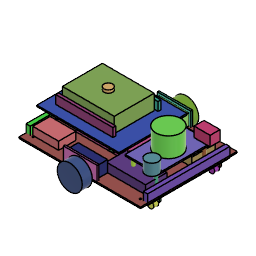
Vibration_Aware_AMR_Concept_v02 (Autodesk Fusion 360 design; units mm, degrees)
part number: 2026-07-23-00-14-06-650
part number: 2026-07-23-00-14-06-952
part number: 2026-07-23-00-14-07-093
part number: 2026-07-23-00-14-07-134
part number: 2026-07-23-00-14-07-172
part number: 2026-07-23-00-14-07-216
part number: 2026-07-23-00-14-07-265
part number: 2026-07-23-00-14-07-312
part number: 2026-07-23-00-14-07-363
part number: 2026-07-23-00-14-07-419
part number: 2026-07-23-00-14-07-476
part number: 2026-07-23-00-14-07-530
part number: 2026-07-23-00-14-07-582
part number: 2026-07-23-00-14-07-638
part number: 2026-07-23-00-14-07-701
part number: 2026-07-23-00-14-07-770
part number: 2026-07-23-00-14-07-834
part number: 2026-07-23-00-14-07-909
part number: 2026-07-23-00-14-07-976
part number: 2026-07-23-00-14-08-046
part number: 2026-07-23-00-14-08-123
part number: 2026-07-23-00-14-08-206
part number: 2026-07-23-00-14-08-287
part number: 2026-07-23-00-14-08-375
part number: 2026-07-23-00-14-08-464
part number: 2026-07-23-00-14-08-554
part number: 2026-07-23-00-14-08-651
part number: 2026-07-23-00-14-08-745
part number: 2026-07-23-00-14-08-842
part number: 2026-07-23-00-14-08-938
part number: 2026-07-23-00-14-09-021
part number: 2026-07-23-00-14-09-105
part number: 2026-07-23-00-14-09-197
part number: 2026-07-23-00-14-09-296
part number: 2026-07-23-00-14-09-389
part number: 2026-07-23-00-14-09-480
part number: 2026-07-23-00-14-09-570
part number: 2026-07-23-00-14-09-668
part number: 2026-07-23-00-14-09-762
part number: 2026-07-23-00-14-09-860
part number: 2026-07-23-00-14-09-959
part number: 2026-07-23-00-14-10-055
part number: 2026-07-23-00-14-10-157
Autodesk Fusion 360 part; units mm, degrees
sketch "00_Chassis_Base_Plate_Footprint" plane through (0, 0, 0) normal (0, 0, 1) x (1, 0, 0) in component "00_Chassis_Base_Plate"
  line L0 (-170, -135) -> (170, -135)
  line L1 (170, -135) -> (170, 135)
  line L2 (170, 135) -> (-170, 135)
  line L3 (-170, 135) -> (-170, -135)
extrude "00_Chassis_Base_Plate_Extrude" add sketch "00_Chassis_Base_Plate_Footprint" along normal blind 4 makes body 1 in component "00_Chassis_Base_Plate"
sketch "Mounting_Hole_Grid" plane through (0, 0, 0) normal (0, 0, 1) x (1, 0, 0) in component "00_Chassis_Base_Plate"
  circle A0 centre (-150, -115) radius 2.5
  circle A1 centre (-150, 115) radius 2.5
  circle A2 centre (150, -115) radius 2.5
  circle A3 centre (150, 115) radius 2.5
  circle A4 centre (-100, -85) radius 2.5
  circle A5 centre (-100, 85) radius 2.5
  circle A6 centre (0, -85) radius 2.5
  circle A7 centre (0, 85) radius 2.5
  circle A8 centre (100, -85) radius 2.5
  circle A9 centre (100, 85) radius 2.5
extrude "Mounting_Holes_Cut" cut sketch "Mounting_Hole_Grid" along normal blind 4 bodies 1 in component "00_Chassis_Base_Plate"
sketch "01_Left_Drive_Wheel_Profile" plane through (0, 0, 0) normal (0, 1, 0) x (1, 0, 0) in component "01_Left_Drive_Wheel"
  circle A0 centre (0, 0) radius 35
extrude "01_Left_Drive_Wheel_Extrude" add sketch "01_Left_Drive_Wheel_Profile" along normal blind 28 separate body makes body 2 in component "01_Left_Drive_Wheel"
sketch "02_Right_Drive_Wheel_Profile" plane through (0, 0, 0) normal (0, 1, 0) x (1, 0, 0) in component "02_Right_Drive_Wheel"
  circle A0 centre (0, 0) radius 35
extrude "02_Right_Drive_Wheel_Extrude" add sketch "02_Right_Drive_Wheel_Profile" along normal blind 28 separate body makes body 3 in component "02_Right_Drive_Wheel"
sketch "03_Left_Wheel_Guard_Footprint" plane through (0, 0, 0) normal (0, 0, 1) x (1, 0, 0) in component "03_Left_Wheel_Guard"
  line L0 (-47, -2.5) -> (47, -2.5)
  line L1 (47, -2.5) -> (47, 2.5)
  line L2 (47, 2.5) -> (-47, 2.5)
  line L3 (-47, 2.5) -> (-47, -2.5)
extrude "03_Left_Wheel_Guard_Extrude" add sketch "03_Left_Wheel_Guard_Footprint" along normal blind 42 separate body makes body 4 in component "03_Left_Wheel_Guard"
sketch "04_Right_Wheel_Guard_Footprint" plane through (0, 0, 0) normal (0, 0, 1) x (1, 0, 0) in component "04_Right_Wheel_Guard"
  line L0 (-47, -2.5) -> (47, -2.5)
  line L1 (47, -2.5) -> (47, 2.5)
  line L2 (47, 2.5) -> (-47, 2.5)
  line L3 (-47, 2.5) -> (-47, -2.5)
extrude "04_Right_Wheel_Guard_Extrude" add sketch "04_Right_Wheel_Guard_Footprint" along normal blind 42 separate body makes body 5 in component "04_Right_Wheel_Guard"
sketch "05_Rear_Caster_Soft_Tread_Profile" plane through (0, 0, 0) normal (0, 1, 0) x (1, 0, 0) in component "05_Rear_Caster_Soft_Tread"
  circle A0 centre (0, 0) radius 20
extrude "05_Rear_Caster_Soft_Tread_Extrude" add sketch "05_Rear_Caster_Soft_Tread_Profile" along normal blind 24 separate body makes body 6 in component "05_Rear_Caster_Soft_Tread"
sketch "06_Rear_Caster_Fork_Left_Footprint" plane through (0, 0, 0) normal (0, 0, 1) x (1, 0, 0) in component "06_Rear_Caster_Fork_Left"
  line L0 (-21, -2) -> (21, -2)
  line L1 (21, -2) -> (21, 2)
  line L2 (21, 2) -> (-21, 2)
  line L3 (-21, 2) -> (-21, -2)
extrude "06_Rear_Caster_Fork_Left_Extrude" add sketch "06_Rear_Caster_Fork_Left_Footprint" along normal blind 26 separate body makes body 7 in component "06_Rear_Caster_Fork_Left"
sketch "07_Rear_Caster_Fork_Right_Footprint" plane through (0, 0, 0) normal (0, 0, 1) x (1, 0, 0) in component "07_Rear_Caster_Fork_Right"
  line L0 (-21, -2) -> (21, -2)
  line L1 (21, -2) -> (21, 2)
  line L2 (21, 2) -> (-21, 2)
  line L3 (-21, 2) -> (-21, -2)
extrude "07_Rear_Caster_Fork_Right_Extrude" add sketch "07_Rear_Caster_Fork_Right_Footprint" along normal blind 26 separate body makes body 8 in component "07_Rear_Caster_Fork_Right"
sketch "08_Rear_Caster_Fork_Bridge_Footprint" plane through (0, 0, 0) normal (0, 0, 1) x (1, 0, 0) in component "08_Rear_Caster_Fork_Bridge"
  line L0 (-14, -19) -> (14, -19)
  line L1 (14, -19) -> (14, 19)
  line L2 (14, 19) -> (-14, 19)
  line L3 (-14, 19) -> (-14, -19)
extrude "08_Rear_Caster_Fork_Bridge_Extrude" add sketch "08_Rear_Caster_Fork_Bridge_Footprint" along normal blind 5 separate body makes body 9 in component "08_Rear_Caster_Fork_Bridge"
sketch "09_Rear_Caster_Swivel_Stem_Profile" plane through (0, 0, 0) normal (0, 0, 1) x (1, 0, 0) in component "09_Rear_Caster_Swivel_Stem"
  circle A0 centre (0, 0) radius 8
extrude "09_Rear_Caster_Swivel_Stem_Extrude" add sketch "09_Rear_Caster_Swivel_Stem_Profile" along normal blind 10 separate body makes body 10 in component "09_Rear_Caster_Swivel_Stem"
sketch "10_Front_AntiTip_Roller_Left_Profile" plane through (0, 0, 0) normal (0, 1, 0) x (1, 0, 0) in component "10_Front_AntiTip_Roller_Left"
  circle A0 centre (0, 0) radius 10
extrude "10_Front_AntiTip_Roller_Left_Extrude" add sketch "10_Front_AntiTip_Roller_Left_Profile" along normal blind 14 separate body makes body 11 in component "10_Front_AntiTip_Roller_Left"
sketch "11_Front_AntiTip_Roller_Right_Profile" plane through (0, 0, 0) normal (0, 1, 0) x (1, 0, 0) in component "11_Front_AntiTip_Roller_Right"
  circle A0 centre (0, 0) radius 10
extrude "11_Front_AntiTip_Roller_Right_Extrude" add sketch "11_Front_AntiTip_Roller_Right_Profile" along normal blind 14 separate body makes body 12 in component "11_Front_AntiTip_Roller_Right"
sketch "12_Front_AntiTip_Bracket_Left_Footprint" plane through (0, 0, 0) normal (0, 0, 1) x (1, 0, 0) in component "12_Front_AntiTip_Bracket_Left"
  line L0 (-17, -2.5) -> (17, -2.5)
  line L1 (17, -2.5) -> (17, 2.5)
  line L2 (17, 2.5) -> (-17, 2.5)
  line L3 (-17, 2.5) -> (-17, -2.5)
extrude "12_Front_AntiTip_Bracket_Left_Extrude" add sketch "12_Front_AntiTip_Bracket_Left_Footprint" along normal blind 18 separate body makes body 13 in component "12_Front_AntiTip_Bracket_Left"
sketch "13_Front_AntiTip_Bracket_Right_Footprint" plane through (0, 0, 0) normal (0, 0, 1) x (1, 0, 0) in component "13_Front_AntiTip_Bracket_Right"
  line L0 (-17, -2.5) -> (17, -2.5)
  line L1 (17, -2.5) -> (17, 2.5)
  line L2 (17, 2.5) -> (-17, 2.5)
  line L3 (-17, 2.5) -> (-17, -2.5)
extrude "13_Front_AntiTip_Bracket_Right_Extrude" add sketch "13_Front_AntiTip_Bracket_Right_Footprint" along normal blind 18 separate body makes body 14 in component "13_Front_AntiTip_Bracket_Right"
sketch "20_Left_Gearmotor_Envelope_Footprint" plane through (0, 0, 0) normal (0, 0, 1) x (1, 0, 0) in component "20_Left_Gearmotor_Envelope"
  line L0 (-41, -16) -> (41, -16)
  line L1 (41, -16) -> (41, 16)
  line L2 (41, 16) -> (-41, 16)
  line L3 (-41, 16) -> (-41, -16)
extrude "20_Left_Gearmotor_Envelope_Extrude" add sketch "20_Left_Gearmotor_Envelope_Footprint" along normal blind 32 separate body makes body 15 in component "20_Left_Gearmotor_Envelope"
sketch "21_Right_Gearmotor_Envelope_Footprint" plane through (0, 0, 0) normal (0, 0, 1) x (1, 0, 0) in component "21_Right_Gearmotor_Envelope"
  line L0 (-41, -16) -> (41, -16)
  line L1 (41, -16) -> (41, 16)
  line L2 (41, 16) -> (-41, 16)
  line L3 (-41, 16) -> (-41, -16)
extrude "21_Right_Gearmotor_Envelope_Extrude" add sketch "21_Right_Gearmotor_Envelope_Footprint" along normal blind 32 separate body makes body 16 in component "21_Right_Gearmotor_Envelope"
sketch "22_Low_Central_Battery_12V_Envelope_Footprint" plane through (0, 0, 0) normal (0, 0, 1) x (1, 0, 0) in component "22_Low_Central_Battery_12V_Envelope"
  line L0 (-72.5, -43) -> (72.5, -43)
  line L1 (72.5, -43) -> (72.5, 43)
  line L2 (72.5, 43) -> (-72.5, 43)
  line L3 (-72.5, 43) -> (-72.5, -43)
extrude "22_Low_Central_Battery_12V_Envelope_Extrude" add sketch "22_Low_Central_Battery_12V_Envelope_Footprint" along normal blind 42 separate body makes body 17 in component "22_Low_Central_Battery_12V_Envelope"
sketch "23_Battery_Retention_Crossbar_Footprint" plane through (0, 0, 0) normal (0, 0, 1) x (1, 0, 0) in component "23_Battery_Retention_Crossbar"
  line L0 (-6, -50) -> (6, -50)
  line L1 (6, -50) -> (6, 50)
  line L2 (6, 50) -> (-6, 50)
  line L3 (-6, 50) -> (-6, -50)
extrude "23_Battery_Retention_Crossbar_Extrude" add sketch "23_Battery_Retention_Crossbar_Footprint" along normal blind 12 separate body makes body 18 in component "23_Battery_Retention_Crossbar"
sketch "24_Raspberry_Pi_4_Envelope_Footprint" plane through (0, 0, 0) normal (0, 0, 1) x (1, 0, 0) in component "24_Raspberry_Pi_4_Envelope"
  line L0 (-45, -32.5) -> (45, -32.5)
  line L1 (45, -32.5) -> (45, 32.5)
  line L2 (45, 32.5) -> (-45, 32.5)
  line L3 (-45, 32.5) -> (-45, -32.5)
extrude "24_Raspberry_Pi_4_Envelope_Extrude" add sketch "24_Raspberry_Pi_4_Envelope_Footprint" along normal blind 24 separate body makes body 19 in component "24_Raspberry_Pi_4_Envelope"
sketch "25_Arduino_Mega_Envelope_Footprint" plane through (0, 0, 0) normal (0, 0, 1) x (1, 0, 0) in component "25_Arduino_Mega_Envelope"
  line L0 (-55, -30) -> (55, -30)
  line L1 (55, -30) -> (55, 30)
  line L2 (55, 30) -> (-55, 30)
  line L3 (-55, 30) -> (-55, -30)
extrude "25_Arduino_Mega_Envelope_Extrude" add sketch "25_Arduino_Mega_Envelope_Footprint" along normal blind 24 separate body makes body 20 in component "25_Arduino_Mega_Envelope"
sketch "26_Motor_Driver_Envelope_Footprint" plane through (0, 0, 0) normal (0, 0, 1) x (1, 0, 0) in component "26_Motor_Driver_Envelope"
  line L0 (-36, -26) -> (36, -26)
  line L1 (36, -26) -> (36, 26)
  line L2 (36, 26) -> (-36, 26)
  line L3 (-36, 26) -> (-36, -26)
extrude "26_Motor_Driver_Envelope_Extrude" add sketch "26_Motor_Driver_Envelope_Footprint" along normal blind 22 separate body makes body 21 in component "26_Motor_Driver_Envelope"
sketch "27_Power_Distribution_Envelope_Footprint" plane through (0, 0, 0) normal (0, 0, 1) x (1, 0, 0) in component "27_Power_Distribution_Envelope"
  line L0 (-36, -24) -> (36, -24)
  line L1 (36, -24) -> (36, 24)
  line L2 (36, 24) -> (-36, 24)
  line L3 (-36, 24) -> (-36, -24)
extrude "27_Power_Distribution_Envelope_Extrude" add sketch "27_Power_Distribution_Envelope_Footprint" along normal blind 22 separate body makes body 22 in component "27_Power_Distribution_Envelope"
sketch "28_Chassis_IMU_Envelope_Profile" plane through (0, 0, 0) normal (0, 0, 1) x (1, 0, 0) in component "28_Chassis_IMU_Envelope"
  circle A0 centre (0, 0) radius 12
extrude "28_Chassis_IMU_Envelope_Extrude" add sketch "28_Chassis_IMU_Envelope_Profile" along normal blind 8 separate body makes body 23 in component "28_Chassis_IMU_Envelope"
sketch "30_Sensor_Bridge_Standoff_1_Profile" plane through (0, 0, 0) normal (0, 0, 1) x (1, 0, 0) in component "30_Sensor_Bridge_Standoff_1"
  circle A0 centre (0, 0) radius 5
extrude "30_Sensor_Bridge_Standoff_1_Extrude" add sketch "30_Sensor_Bridge_Standoff_1_Profile" along normal blind 42 separate body makes body 24 in component "30_Sensor_Bridge_Standoff_1"
sketch "30_Sensor_Bridge_Standoff_2_Profile" plane through (0, 0, 0) normal (0, 0, 1) x (1, 0, 0) in component "30_Sensor_Bridge_Standoff_2"
  circle A0 centre (0, 0) radius 5
extrude "30_Sensor_Bridge_Standoff_2_Extrude" add sketch "30_Sensor_Bridge_Standoff_2_Profile" along normal blind 42 separate body makes body 25 in component "30_Sensor_Bridge_Standoff_2"
sketch "30_Sensor_Bridge_Standoff_3_Profile" plane through (0, 0, 0) normal (0, 0, 1) x (1, 0, 0) in component "30_Sensor_Bridge_Standoff_3"
  circle A0 centre (0, 0) radius 5
extrude "30_Sensor_Bridge_Standoff_3_Extrude" add sketch "30_Sensor_Bridge_Standoff_3_Profile" along normal blind 42 separate body makes body 26 in component "30_Sensor_Bridge_Standoff_3"
sketch "30_Sensor_Bridge_Standoff_4_Profile" plane through (0, 0, 0) normal (0, 0, 1) x (1, 0, 0) in component "30_Sensor_Bridge_Standoff_4"
  circle A0 centre (0, 0) radius 5
extrude "30_Sensor_Bridge_Standoff_4_Extrude" add sketch "30_Sensor_Bridge_Standoff_4_Profile" along normal blind 42 separate body makes body 27 in component "30_Sensor_Bridge_Standoff_4"
sketch "34_Rigid_Sensor_Bridge_Footprint" plane through (0, 0, 0) normal (0, 0, 1) x (1, 0, 0) in component "34_Rigid_Sensor_Bridge"
  line L0 (-46, -75) -> (46, -75)
  line L1 (46, -75) -> (46, 75)
  line L2 (46, 75) -> (-46, 75)
  line L3 (-46, 75) -> (-46, -75)
extrude "34_Rigid_Sensor_Bridge_Extrude" add sketch "34_Rigid_Sensor_Bridge_Footprint" along normal blind 4 separate body makes body 28 in component "34_Rigid_Sensor_Bridge"
sketch "35_RPLIDAR_A1_Rigid_Envelope_Profile" plane through (0, 0, 0) normal (0, 0, 1) x (1, 0, 0) in component "35_RPLIDAR_A1_Rigid_Envelope"
  circle A0 centre (0, 0) radius 35
extrude "35_RPLIDAR_A1_Rigid_Envelope_Extrude" add sketch "35_RPLIDAR_A1_Rigid_Envelope_Profile" along normal blind 55 separate body makes body 29 in component "35_RPLIDAR_A1_Rigid_Envelope"
sketch "36_USB_Camera_Rigid_Envelope_Footprint" plane through (0, 0, 0) normal (0, 0, 1) x (1, 0, 0) in component "36_USB_Camera_Rigid_Envelope"
  line L0 (-22.5, -14) -> (22.5, -14)
  line L1 (22.5, -14) -> (22.5, 14)
  line L2 (22.5, 14) -> (-22.5, 14)
  line L3 (-22.5, 14) -> (-22.5, -14)
extrude "36_USB_Camera_Rigid_Envelope_Extrude" add sketch "36_USB_Camera_Rigid_Envelope_Footprint" along normal blind 28 separate body makes body 30 in component "36_USB_Camera_Rigid_Envelope"
sketch "37_Emergency_Stop_Envelope_Profile" plane through (0, 0, 0) normal (0, 0, 1) x (1, 0, 0) in component "37_Emergency_Stop_Envelope"
  circle A0 centre (0, 0) radius 18
extrude "37_Emergency_Stop_Envelope_Extrude" add sketch "37_Emergency_Stop_Envelope_Profile" along normal blind 32 separate body makes body 31 in component "37_Emergency_Stop_Envelope"
sketch "40_Elastomer_Isolator_1_Profile" plane through (0, 0, 0) normal (0, 0, 1) x (1, 0, 0) in component "40_Elastomer_Isolator_1"
  circle A0 centre (0, 0) radius 12
extrude "40_Elastomer_Isolator_1_Extrude" add sketch "40_Elastomer_Isolator_1_Profile" along normal blind 16 separate body makes body 32 in component "40_Elastomer_Isolator_1"
sketch "40_Elastomer_Isolator_2_Profile" plane through (0, 0, 0) normal (0, 0, 1) x (1, 0, 0) in component "40_Elastomer_Isolator_2"
  circle A0 centre (0, 0) radius 12
extrude "40_Elastomer_Isolator_2_Extrude" add sketch "40_Elastomer_Isolator_2_Profile" along normal blind 16 separate body makes body 33 in component "40_Elastomer_Isolator_2"
sketch "40_Elastomer_Isolator_3_Profile" plane through (0, 0, 0) normal (0, 0, 1) x (1, 0, 0) in component "40_Elastomer_Isolator_3"
  circle A0 centre (0, 0) radius 12
extrude "40_Elastomer_Isolator_3_Extrude" add sketch "40_Elastomer_Isolator_3_Profile" along normal blind 16 separate body makes body 34 in component "40_Elastomer_Isolator_3"
sketch "40_Elastomer_Isolator_4_Profile" plane through (0, 0, 0) normal (0, 0, 1) x (1, 0, 0) in component "40_Elastomer_Isolator_4"
  circle A0 centre (0, 0) radius 12
extrude "40_Elastomer_Isolator_4_Extrude" add sketch "40_Elastomer_Isolator_4_Profile" along normal blind 16 separate body makes body 35 in component "40_Elastomer_Isolator_4"
sketch "44_Isolated_Payload_Deck_Footprint" plane through (0, 0, 0) normal (0, 0, 1) x (1, 0, 0) in component "44_Isolated_Payload_Deck"
  line L0 (-115, -95) -> (115, -95)
  line L1 (115, -95) -> (115, 95)
  line L2 (115, 95) -> (-115, 95)
  line L3 (-115, 95) -> (-115, -95)
extrude "44_Isolated_Payload_Deck_Extrude" add sketch "44_Isolated_Payload_Deck_Footprint" along normal blind 4 separate body makes body 36 in component "44_Isolated_Payload_Deck"
sketch "45_Fragile_Payload_Envelope_Footprint" plane through (0, 0, 0) normal (0, 0, 1) x (1, 0, 0) in component "45_Fragile_Payload_Envelope"
  line L0 (-72.5, -56) -> (72.5, -56)
  line L1 (72.5, -56) -> (72.5, 56)
  line L2 (72.5, 56) -> (-72.5, 56)
  line L3 (-72.5, 56) -> (-72.5, -56)
extrude "45_Fragile_Payload_Envelope_Extrude" add sketch "45_Fragile_Payload_Envelope_Footprint" along normal blind 42 separate body makes body 37 in component "45_Fragile_Payload_Envelope"
sketch "46_Payload_Retention_Rail_Left_Footprint" plane through (0, 0, 0) normal (0, 0, 1) x (1, 0, 0) in component "46_Payload_Retention_Rail_Left"
  line L0 (-80, -4) -> (80, -4)
  line L1 (80, -4) -> (80, 4)
  line L2 (80, 4) -> (-80, 4)
  line L3 (-80, 4) -> (-80, -4)
extrude "46_Payload_Retention_Rail_Left_Extrude" add sketch "46_Payload_Retention_Rail_Left_Footprint" along normal blind 24 separate body makes body 38 in component "46_Payload_Retention_Rail_Left"
sketch "47_Payload_Retention_Rail_Right_Footprint" plane through (0, 0, 0) normal (0, 0, 1) x (1, 0, 0) in component "47_Payload_Retention_Rail_Right"
  line L0 (-80, -4) -> (80, -4)
  line L1 (80, -4) -> (80, 4)
  line L2 (80, 4) -> (-80, 4)
  line L3 (-80, 4) -> (-80, -4)
extrude "47_Payload_Retention_Rail_Right_Extrude" add sketch "47_Payload_Retention_Rail_Right_Footprint" along normal blind 24 separate body makes body 39 in component "47_Payload_Retention_Rail_Right"
sketch "48_Payload_IMU_Envelope_Profile" plane through (0, 0, 0) normal (0, 0, 1) x (1, 0, 0) in component "48_Payload_IMU_Envelope"
  circle A0 centre (0, 0) radius 12
extrude "48_Payload_IMU_Envelope_Extrude" add sketch "48_Payload_IMU_Envelope_Profile" along normal blind 8 separate body makes body 40 in component "48_Payload_IMU_Envelope"
sketch "50_Front_Energy_Absorbing_Bumper_Footprint" plane through (0, 0, 0) normal (0, 0, 1) x (1, 0, 0) in component "50_Front_Energy_Absorbing_Bumper"
  line L0 (-6, -115) -> (6, -115)
  line L1 (6, -115) -> (6, 115)
  line L2 (6, 115) -> (-6, 115)
  line L3 (-6, 115) -> (-6, -115)
extrude "50_Front_Energy_Absorbing_Bumper_Extrude" add sketch "50_Front_Energy_Absorbing_Bumper_Footprint" along normal blind 28 separate body makes body 41 in component "50_Front_Energy_Absorbing_Bumper"
sketch "51_Rear_Energy_Absorbing_Bumper_Footprint" plane through (0, 0, 0) normal (0, 0, 1) x (1, 0, 0) in component "51_Rear_Energy_Absorbing_Bumper"
  line L0 (-6, -115) -> (6, -115)
  line L1 (6, -115) -> (6, 115)
  line L2 (6, 115) -> (-6, 115)
  line L3 (-6, 115) -> (-6, -115)
extrude "51_Rear_Energy_Absorbing_Bumper_Extrude" add sketch "51_Rear_Energy_Absorbing_Bumper_Footprint" along normal blind 28 separate body makes body 42 in component "51_Rear_Energy_Absorbing_Bumper"
component "00_Chassis_Base_Plate" placed x (1, 0, 0) y (0, 1, 0) z (0, 0, 1) at (0, 0, 30)
component "01_Left_Drive_Wheel" placed x (1, 0, 0) y (0, 1, 0) z (0, 0, 1) at (0, -163, 35)
component "02_Right_Drive_Wheel" placed x (1, 0, 0) y (0, 1, 0) z (0, 0, 1) at (0, 135, 35)
component "03_Left_Wheel_Guard" placed x (1, 0, 0) y (0, 1, 0) z (0, 0, 1) at (0, -131, 31)
component "04_Right_Wheel_Guard" placed x (1, 0, 0) y (0, 1, 0) z (0, 0, 1) at (0, 131, 31)
component "05_Rear_Caster_Soft_Tread" placed x (1, 0, 0) y (0, 1, 0) z (0, 0, 1) at (-132, -12, 20)
component "06_Rear_Caster_Fork_Left" placed x (1, 0, 0) y (0, 1, 0) z (0, 0, 1) at (-132, -17, 20)
component "07_Rear_Caster_Fork_Right" placed x (1, 0, 0) y (0, 1, 0) z (0, 0, 1) at (-132, 17, 20)
component "08_Rear_Caster_Fork_Bridge" placed x (1, 0, 0) y (0, 1, 0) z (0, 0, 1) at (-132, 0, 43)
component "09_Rear_Caster_Swivel_Stem" placed x (1, 0, 0) y (0, 1, 0) z (0, 0, 1) at (-132, 0, 48)
component "10_Front_AntiTip_Roller_Left" placed x (1, 0, 0) y (0, 1, 0) z (0, 0, 1) at (154, -92, 11)
component "11_Front_AntiTip_Roller_Right" placed x (1, 0, 0) y (0, 1, 0) z (0, 0, 1) at (154, 78, 11)
component "12_Front_AntiTip_Bracket_Left" placed x (1, 0, 0) y (0, 1, 0) z (0, 0, 1) at (150, -77, 16)
component "13_Front_AntiTip_Bracket_Right" placed x (1, 0, 0) y (0, 1, 0) z (0, 0, 1) at (150, 92, 16)
component "20_Left_Gearmotor_Envelope" placed x (1, 0, 0) y (0, 1, 0) z (0, 0, 1) at (0, -114, 34)
component "21_Right_Gearmotor_Envelope" placed x (1, 0, 0) y (0, 1, 0) z (0, 0, 1) at (0, 114, 34)
component "22_Low_Central_Battery_12V_Envelope" placed x (1, 0, 0) y (0, 1, 0) z (0, 0, 1) at (-30, 0, 34)
component "23_Battery_Retention_Crossbar" placed x (1, 0, 0) y (0, 1, 0) z (0, 0, 1) at (-30, 0, 72)
component "24_Raspberry_Pi_4_Envelope" placed x (1, 0, 0) y (0, 1, 0) z (0, 0, 1) at (100, 66, 34)
component "25_Arduino_Mega_Envelope" placed x (1, 0, 0) y (0, 1, 0) z (0, 0, 1) at (92, -68, 34)
component "26_Motor_Driver_Envelope" placed x (1, 0, 0) y (0, 1, 0) z (0, 0, 1) at (-118, 86, 34)
component "27_Power_Distribution_Envelope" placed x (1, 0, 0) y (0, 1, 0) z (0, 0, 1) at (-118, -88, 34)
component "28_Chassis_IMU_Envelope" placed x (1, 0, 0) y (0, 1, 0) z (0, 0, 1) at (58, 0, 34)
component "30_Sensor_Bridge_Standoff_1" placed x (1, 0, 0) y (0, 1, 0) z (0, 0, 1) at (82, -67, 34)
component "30_Sensor_Bridge_Standoff_2" placed x (1, 0, 0) y (0, 1, 0) z (0, 0, 1) at (82, 67, 34)
component "30_Sensor_Bridge_Standoff_3" placed x (1, 0, 0) y (0, 1, 0) z (0, 0, 1) at (145, -67, 34)
component "30_Sensor_Bridge_Standoff_4" placed x (1, 0, 0) y (0, 1, 0) z (0, 0, 1) at (145, 67, 34)
component "34_Rigid_Sensor_Bridge" placed x (1, 0, 0) y (0, 1, 0) z (0, 0, 1) at (113, 0, 76)
component "35_RPLIDAR_A1_Rigid_Envelope" placed x (1, 0, 0) y (0, 1, 0) z (0, 0, 1) at (113, 0, 80)
component "36_USB_Camera_Rigid_Envelope" placed x (1, 0, 0) y (0, 1, 0) z (0, 0, 1) at (145, 76, 80)
component "37_Emergency_Stop_Envelope" placed x (1, 0, 0) y (0, 1, 0) z (0, 0, 1) at (145, -78, 80)
component "40_Elastomer_Isolator_1" placed x (1, 0, 0) y (0, 1, 0) z (0, 0, 1) at (-125, -72, 76)
component "40_Elastomer_Isolator_2" placed x (1, 0, 0) y (0, 1, 0) z (0, 0, 1) at (-125, 72, 76)
component "40_Elastomer_Isolator_3" placed x (1, 0, 0) y (0, 1, 0) z (0, 0, 1) at (35, -72, 76)
component "40_Elastomer_Isolator_4" placed x (1, 0, 0) y (0, 1, 0) z (0, 0, 1) at (35, 72, 76)
component "44_Isolated_Payload_Deck" placed x (1, 0, 0) y (0, 1, 0) z (0, 0, 1) at (-45, 0, 92)
component "45_Fragile_Payload_Envelope" placed x (1, 0, 0) y (0, 1, 0) z (0, 0, 1) at (-55, 0, 96)
component "46_Payload_Retention_Rail_Left" placed x (1, 0, 0) y (0, 1, 0) z (0, 0, 1) at (-55, -63, 96)
component "47_Payload_Retention_Rail_Right" placed x (1, 0, 0) y (0, 1, 0) z (0, 0, 1) at (-55, 63, 96)
component "48_Payload_IMU_Envelope" placed x (1, 0, 0) y (0, 1, 0) z (0, 0, 1) at (-55, 0, 138)
component "50_Front_Energy_Absorbing_Bumper" placed x (1, 0, 0) y (0, 1, 0) z (0, 0, 1) at (164, 0, 28)
component "51_Rear_Energy_Absorbing_Bumper" placed x (1, 0, 0) y (0, 1, 0) z (0, 0, 1) at (-164, 0, 28)
equation "chassisLength = 340 mm" comment "Provisional overall base-plate length"
equation "chassisWidth = 270 mm" comment "Provisional overall base-plate width"
equation "baseThickness = 4 mm" comment "Prototype plate thickness"
equation "wheelDiameter = 70 mm" comment "Placeholder drive-wheel diameter"
equation "wheelWidth = 28 mm" comment "Placeholder drive-wheel width"
equation "driveTrackWidth = 298 mm" comment "Outside-to-outside provisional drive-wheel track"
equation "casterDiameter = 40 mm" comment "Soft-tread rear caster clearance envelope"
equation "payloadDeckHeight = 92 mm" comment "Top of isolated payload deck above ground datum"
equation "payloadDeckLength = 230 mm" comment "Isolated payload-deck length"
equation "payloadDeckWidth = 190 mm" comment "Isolated payload-deck width"
equation "isolatorHeight = 16 mm" comment "Provisional elastomer isolator height"
equation "lidarDiameter = 70 mm" comment "RPLIDAR A1 clearance envelope"
equation "payloadMassTarget = 1500 g" comment "Provisional representative payload limit"
named bodies: "00_Chassis_Base_Plate", "01_Left_Drive_Wheel", "02_Right_Drive_Wheel", "03_Left_Wheel_Guard", "04_Right_Wheel_Guard", "05_Rear_Caster_Soft_Tread", "06_Rear_Caster_Fork_Left", "07_Rear_Caster_Fork_Right", "08_Rear_Caster_Fork_Bridge", "09_Rear_Caster_Swivel_Stem", "10_Front_AntiTip_Roller_Left", "11_Front_AntiTip_Roller_Right", "12_Front_AntiTip_Bracket_Left", "13_Front_AntiTip_Bracket_Right", "20_Left_Gearmotor_Envelope", "21_Right_Gearmotor_Envelope", "22_Low_Central_Battery_12V_Envelope", "23_Battery_Retention_Crossbar", "24_Raspberry_Pi_4_Envelope", "25_Arduino_Mega_Envelope", "26_Motor_Driver_Envelope", "27_Power_Distribution_Envelope", "28_Chassis_IMU_Envelope", "30_Sensor_Bridge_Standoff_1", "30_Sensor_Bridge_Standoff_2", "30_Sensor_Bridge_Standoff_3", "30_Sensor_Bridge_Standoff_4", "34_Rigid_Sensor_Bridge", "35_RPLIDAR_A1_Rigid_Envelope", "36_USB_Camera_Rigid_Envelope", "37_Emergency_Stop_Envelope", "40_Elastomer_Isolator_1", "40_Elastomer_Isolator_2", "40_Elastomer_Isolator_3", "40_Elastomer_Isolator_4", "44_Isolated_Payload_Deck", "45_Fragile_Payload_Envelope", "46_Payload_Retention_Rail_Left", "47_Payload_Retention_Rail_Right", "48_Payload_IMU_Envelope", "50_Front_Energy_Absorbing_Bumper", "51_Rear_Energy_Absorbing_Bumper"
